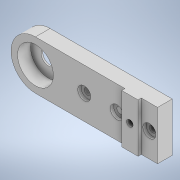
# Autodesk Inventor part: bearing_mount
Saved by Autodesk Inventor 2022 (Build 260153000, 153)
## iProperties
Created: 2022-01-28
Part Number: bearing_mount
Material: Generic
Document SubType Name: Modeling
Designer: Martijn
Density: 1 g/cm^3
Appearance: Default
Author: Martijn
Autodesk Inventor part; units mm, degrees
ref_plane "YZ Plane" through (0, 0, 0) normal (1, 0, 0) x (0, 1, 0)
ref_plane "XZ Plane" through (0, 0, 0) normal (0, 1, 0) x (-1, 0, 0)
ref_plane "XY Plane" through (0, 0, 0) normal (0, 0, 1) x (1, 0, 0)
sketch "Sketch1" plane through (0, 0, 0) normal (0, 0, 1) x (1, 0, 0)
  line L0 (15, 15) -> (90, 15)
  line L1 (90, 15) -> (90, -15)
  line L2 (90, -15) -> (15, -15)
  line L3 (-18, 0) -> (108, 0) projected
  arc A0 (15, 15) -> (15, -15) centre (15, 0) ccw
  line L4 (0, -21) -> (0, 21) projected
  line L5 (15, 0) -> (90, 0)
  point P0 (0, 0)
  dimension "d4" = 30
  dimension "d15" = 15
  dimension "d16" = 75
  constraints: 8 end point, 2 parallel, 2 point on circle, 1 centre point, 1 midpoint, 1 perpendicular, 1 point on line, 1 tangent, 1 vertical
  measures "d4" distance between parallel lines of L2 L0
  measures "d15" radius of A0
  measures "d16" distance from line of L1 L5.start
extrude "Extrusion1" add sketch "Sketch1" along normal blind 9
sketch "Sketch2" plane through (0, 0, 9) normal (0, 0, 1) x (1, 0, 0)
  circle A0 centre (15, 0) radius 11
  arc A1 (15, 15) -> (15, -15) centre (15, 0) ccw projected
  point P0 (0, 0)
  dimension "d7" = 22
  constraints: 1 centre point, 1 concentric
  measures "d7" diameter of A0
extrude "Extrusion2" cut sketch "Sketch2" against normal blind 10
sketch "Sketch3" plane through (0, 0, 9) normal (0, 0, 1) x (1, 0, 0)
  circle A0 centre (65, 0) radius 2
  circle A1 centre (85, 0) radius 2
  line L0 (90, -15) -> (90, 15) projected
  circle A2 centre (45, 0) radius 2
  point P0 (0, 0)
  dimension "d10" = 4
  dimension "d11" = 5
  dimension "d12" = 25
  dimension "d26" = 4
  dimension "d27" = 20
  constraints: 3 centre point, 1 equal radius
  measures "d10" diameter of A0
  measures "d11" distance from line of L0 A1.centre
  measures "d12" distance from line of L0 A0.centre
  measures "d26" diameter of A2
  measures "d27" distance of A0.centre A2.centre
extrude "Extrusion3" cut sketch "Sketch3" against normal blind 25
sketch "Sketch4" plane through (0, 0, 0) normal (0, 0, -1) x (-1, 0, 0)
  circle A0 centre (-15, 0) radius 15
  arc A1 (-15, -15) -> (-15, 15) centre (-15, 0) ccw projected
  circle A2 centre (-15, 0) radius 11 projected
  point P0 (0, 0)
  constraints: 2 concentric, 1 centre point
extrude "Extrusion4" add sketch "Sketch4" against normal blind 1 contours A0 | A2
sketch "Sketch6" plane through (0, 0, 9) normal (0, 0, 1) x (1, 0, 0)
  circle A0 centre (65, 0) radius 2 projected
  circle A1 centre (65, 0) radius 4
  circle A2 centre (85, 0) radius 4
  circle A3 centre (85, 0) radius 2 projected
  circle A4 centre (45, 0) radius 4
  circle A5 centre (45, 0) radius 2 projected
  point P0 (0, 0)
  dimension "d22" = 8
  dimension "d23" = 8
  dimension "d28" = 8
  constraints: 3 centre point, 2 concentric, 1 coincident
  measures "d22" diameter of A1
  measures "d23" diameter of A2
  measures "d28" diameter of A4
extrude "Extrusion6" cut sketch "Sketch6" against normal blind 2
sketch "Sketch7" plane through (0, 0, 0) normal (0, 0, -1) x (-1, 0, 0)
  arc A0 (-15, -15) -> (-15, 15) centre (-15, 0) ccw projected
  circle A1 centre (-15, 0) radius 4.5
  point P0 (0, 0)
  dimension "d29" = 9
  constraints: 1 centre point, 1 coincident
  measures "d29" diameter of A1
extrude "Extrusion7" cut sketch "Sketch7" against normal blind 2
sketch "Sketch8" plane through (0, 0, 9) normal (0, 0, 1) x (1, 0, 0)
  line L0 (90, 15) -> (15, 15) projected
  line L1 (70, 15) -> (80, 15)
  line L2 (80, 15) -> (80, -15)
  line L3 (80, -15) -> (70, -15)
  line L4 (70, -15) -> (70, 15)
  line L5 (90, -15) -> (90, 15) projected
  line L6 (15, -15) -> (90, -15) projected
  point P0 (0, 0)
  dimension "d32" = 10
  dimension "d33" = 10
  constraints: 8 end point, 2 parallel, 1 collinear, 1 horizontal, 1 perpendicular, 1 point on line
  measures "d32" distance between parallel lines of L4 L2
  measures "d33" distance between parallel lines of L5 L2
extrude "Extrusion8" add sketch "Sketch8" along normal blind 2 contours L2 L3 L4 L0
sketch "Sketch9" plane through (0, 0, 11) normal (0, 0, 1) x (1, 0, 0)
  circle A0 centre (75, 0) radius 2
  line L0 (80, -15) -> (80, 15) projected
  line L1 (70, -15) -> (80, -15) projected
  point P0 (0, 0)
  dimension "d36" = 4
  dimension "d37" = 5
  dimension "d38" = 15
  constraints: 1 centre point
  measures "d36" diameter of A0
  measures "d37" distance from line of L0 A0.centre
  measures "d38" distance from line of L1 A0.centre
extrude "Extrusion9" cut sketch "Sketch9" against normal blind 12
equation "\"d13\" = d12"
body "Solid1"
